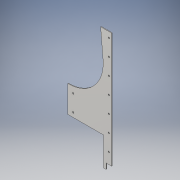
# Autodesk Inventor part: LauncherSidePlateRev2
Saved by Autodesk Inventor 2016 (Build 200138000, 138)
## iProperties
Created: 2017-01-21
Part Number: LauncherSidePlateRev2
Material: Generic
Document SubType Name: Modeling
Designer: madsenn
Density: 1 g/cm^3
Appearance: Default
Author: madsenn
Autodesk Inventor part; units mm, degrees
ref_plane "YZ Plane" through (0, 0, 0) normal (1, 0, 0) x (0, 1, 0)
ref_plane "XZ Plane" through (0, 0, 0) normal (0, 1, 0) x (-1, 0, 0)
ref_plane "XY Plane" through (0, 0, 0) normal (0, 0, 1) x (1, 0, 0)
sketch "Sketch1" plane through (0, 0, 0) normal (0, 0, 1) x (1, 0, 0)
  arc A0 (-2.4847, -161.9059) -> (161.2805, 14.4329) centre (0, 0) ccw
  line L0 (-2.4847, -161.9059) -> (-2.4847, -174.6059)
  line L1 (175.9176, 141.4329) -> (149.9153, 141.4329)
  line L2 (149.9153, 141.4329) -> (200.7153, 141.4329)
  line L3 (200.7153, 141.4329) -> (200.7153, -174.6059)
  line L4 (149.9153, 141.4329) -> (161.2805, 14.4329)
  line L5 (-2.4847, -161.9224) -> (-2.4847, -174.6059)
  line L6 (200.7153, 141.4329) -> (200.7153, -391.7131)
  line L7 (-2.4847, -174.6059) -> (-2.4847, -417.3671)
  line L8 (-2.4847, -417.3671) -> (175.0613, -417.3671)
  line L9 (200.7153, -417.3671) -> (199.9221, -417.3671)
  line L10 (175.0613, -417.3671) -> (175.0613, -391.7131)
  line L11 (175.0613, -391.7131) -> (200.7153, -391.7131)
  dimension "d1" = 323.85
  dimension "d4" = 50.8
  dimension "d6" = 127
  dimension "d9" = 11.3652
  dimension "d10" = 127.5075
  dimension "d11" = 558.8
  dimension "d14" = 203.2
  dimension "d15" = 25.654
  dimension "d16" = 25.654
  constraints: 24 end point, 3 horizontal, 3 perpendicular, 2 point on circle, 2 point on line, 2 vertical, 1 centre point, 1 coincident, 1 collinear, 1 parallel, 1 tangent
  measures "d1" diameter of A0
  measures "d4" distance of L1.end L2.end
  measures "d6" distance from line of L4.end L2
  measures "d9" horizontal distance of L4.end L1.end
  measures "d10" distance of L4.end L1.end
  measures "d11" distance of L2.end L9.start
  measures "d14" distance of L3.end L0.end
  measures "d15" distance of L6.end L10.end
  measures "d16" distance between parallel lines of L8 L11
extrude "Extrusion1" add sketch "Sketch1" along normal blind 3.175
sketch "Sketch2" plane through (0, 0, 3.175) normal (0, 0, 1) x (1, 0, 0)
  line L0 (200.7153, 141.4329) -> (200.7153, -391.7131) projected
  line L1 (200.7153, 141.4329) -> (149.9153, 141.4329) projected
  point P0 (0, 0)
  point P1 (188.0153, 116.0329)
  point P2 (188.0153, 39.8329)
  point P3 (188.0153, -36.3671)
  point P4 (188.0153, -112.5671)
  point P5 (188.0153, -188.7671)
  point P6 (188.0153, -264.9671)
  point P7 (188.0153, -341.1671)
  dimension "d19" = 12.7
  dimension "d20" = 12.7
  dimension "d21" = 12.7
  dimension "d22" = 12.7
  dimension "d23" = 12.7
  dimension "d24" = 12.7
  dimension "d25" = 76.2
  dimension "d26" = 76.2
  dimension "d27" = 76.2
  dimension "d28" = 76.2
  dimension "d29" = 76.2
  dimension "d30" = 76.2
  dimension "d31" = 25.4
  measures "d19" distance from line of L0 point (188.015, 116.033)
  measures "d20" distance from line of L0 point (188.015, 39.833)
  measures "d21" distance from line of L0 point (188.015, -36.367)
  measures "d22" distance from line of L0 point (188.015, -112.567)
  measures "d23" distance from line of L0 point (188.015, -188.767)
  measures "d24" distance from line of L0 point (188.015, -264.967)
  measures "d25" distance of point (188.015, 39.833) point (188.015, 116.033)
  measures "d26" distance of point (188.015, -36.367) point (188.015, 39.833)
  measures "d27" distance of point (188.015, -36.367) point (188.015, -112.567)
  measures "d28" distance of point (188.015, -112.567) point (188.015, -188.767)
  measures "d29" distance of point (188.015, -188.767) point (188.015, -264.967)
  measures "d30" distance of point (188.015, -341.167) point (188.015, -264.967)
  measures "d31" distance from line of L1 point (188.015, 116.033)
hole "Hole1" at (188.0153, 116.0329, 3.175) at (188.0153, 39.8329, 3.175) at (188.0153, -36.3671, 3.175) at (188.0153, -112.5671, 3.175) at (188.0153, -188.7671, 3.175) at (188.0153, -264.9671, 3.175) at (188.0153, -341.1671, 3.175) direction (0, 0, -1) diameter 7.1374 end through all
sketch "Sketch3" plane through (0, 0, 3.175) normal (0, 0, 1) x (1, 0, 0)
  line L0 (-2.4847, -161.9059) -> (-2.4847, -417.3671) projected
  line L1 (-2.4847, -417.3671) -> (175.0613, -417.3671) projected
  point P0 (0, 0)
  point P1 (22.9153, -188.7671)
  point P2 (22.9153, -264.9671)
  point P3 (22.9153, -341.1671)
  dimension "d39" = 25.4
  dimension "d40" = 25.4
  dimension "d41" = 25.4
  dimension "d42" = 76.2
  dimension "d43" = 76.2
  dimension "d44" = 76.2
  measures "d39" distance from line of L0 point (22.915, -188.767)
  measures "d40" distance from line of L0 point (22.915, -264.967)
  measures "d41" distance from line of L0 point (22.915, -341.167)
  measures "d42" distance from line of L1 point (22.915, -341.167)
  measures "d43" distance of point (22.915, -341.167) point (22.915, -264.967)
  measures "d44" distance of point (22.915, -264.967) point (22.915, -188.767)
hole "Hole2" at (22.9153, -188.7671, 3.175) at (22.9153, -264.9671, 3.175) at (22.9153, -341.1671, 3.175) direction (0, 0, -1) diameter 7.1374 end through all
sketch "Sketch4" plane through (0, 0, 3.175) normal (0, 0, 1) x (1, 0, 0)
  line L0 (-2.4847, -417.3671) -> (175.0613, -417.3671) projected
  line L1 (-2.4847, -161.9059) -> (-2.4847, -417.3671) projected
  line L2 (162.6153, -417.3671) -> (-2.4847, -417.3671)
  line L3 (-2.4847, -417.3671) -> (-2.4847, -285.2871)
  line L4 (-2.4847, -285.2871) -> (162.6153, -285.2871)
  line L5 (162.6153, -285.2871) -> (162.6153, -417.3671)
  line L6 (175.0613, -417.3671) -> (175.0613, -391.7131) projected
  line L7 (175.0613, -391.7131) -> (200.7153, -391.7131) projected
  line L8 (200.7153, -391.7131) -> (200.7153, 141.4329) projected
  circle A0 centre (22.9153, -341.1671) radius 3.5687 projected
  circle A1 centre (22.9153, -264.9671) radius 3.5687 projected
  point P0 (0, 0)
  dimension "d52" = 132.08
  dimension "d53" = 38.1
  constraints: 8 end point, 2 parallel, 2 point on line, 1 horizontal, 1 perpendicular
  measures "d52" distance between parallel lines of L0 L4
  measures "d53" distance between parallel lines of L8 L5
extrude "Extrusion2" cut sketch "Sketch4" against normal blind 25.4 contours L1 L4 L5 L0
body "Solid1"
